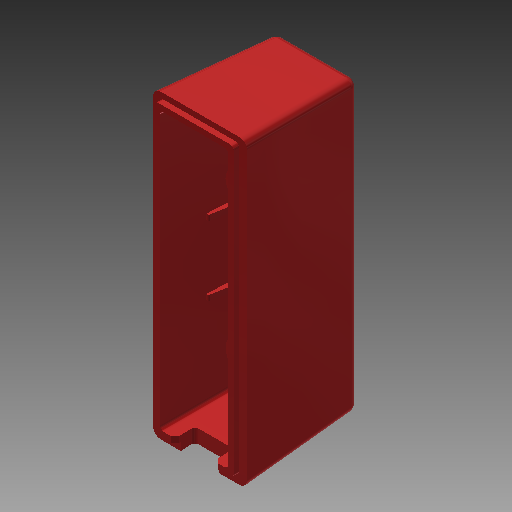
# Autodesk Inventor part: 276-2154
Saved by Autodesk Inventor 2019.4 (Build 234330000, 330)
## iProperties
Category: Sensors
Company: Autodesk Inc.
Created: 2012-03-29
Part Number: 276-2154
Document SubType Name: Modeling
Designer: Autodesk Inc.
Density: 1.06 g/cm^3
Material: ABS Plastic
Catalog Web Link: http://www.vexrobotics.com/276-2154.html
Vendor: VEX
Mass: 3.18655 g
Surface Area: 37.1794 cm^2
Volume: 3.00618 cm^3
Appearance: 浅红色
Author: Autodesk Inc.
Autodesk Inventor part; units mm, degrees
ref_plane "YZ Plane" through (0, 0, 0) normal (1, 0, 0) x (0, 1, 0)
ref_plane "XY Plane" through (0, 0, 0) normal (0, 0, 1) x (1, 0, 0)
sketch "Sketch1" plane through (0, 0, 0) normal (0, 0, 1) x (1, 0, 0)
  line L0 (-1.6366, -1.7521) -> (10.53, -1.7521)
  line L1 (6.89, -1.7521) -> (10.53, -1.7521)
  line L2 (10.53, 37.2479) -> (10.53, -1.7521)
  line L3 (10.53, 37.2479) -> (-1.6366, 37.2479)
  line L4 (-1.6366, 37.2479) -> (-1.6366, -1.7521)
  point P0 (4.4467, 17.7479)
  point P1 (4.4467, 37.2479)
  dimension "d19" = 12.1666
  constraints: 10 end point, 2 horizontal, 1 midpoint, 1 vertical, 1 vertical alignment
  measures "d19" distance between parallel lines of L2 L4
extrude "Extrusion1" add sketch "Sketch1" against normal blind 15.1892 draft -3
fillet "Fillet1" radius 0.9906 8 edges at (-1.2386, 36.8499, -7.5946) (4.4467, -0.956, -15.1892) (-0.8406, 17.7479, -15.1892) (4.4467, 36.4519, -15.1892) (10.132, 36.8499, -7.5946) (9.734, 17.7479, -15.1892) (10.132, -1.354, -7.5946) (-1.2386, -1.354, -7.5946)
sketch "Sketch2" plane through (0, 0, 0) normal (0, 0, 1) x (1, 0, 0)
  line L0 (-0.7514, -1.7426) -> (1.89, -1.7426)
  line L1 (-0.734, -0.7266) -> (-0.734, 36.5367)
  line L2 (-0.734, 36.5367) -> (9.514, 36.5367)
  line L3 (9.514, 36.5367) -> (9.514, -0.7266)
  line L4 (9.514, -0.7266) -> (-0.734, -0.7266)
  line L5 (6.89, -1.7426) -> (9.5314, -1.7426)
  ellipse E0 centre (9.5286, -0.7413) end of major axis (8.8196, -0.0322) minor radius 1 (9.5314, -1.7426) -> (10.53, -0.744) ccw
  line L6 (10.53, 36.2587) -> (10.53, -0.744)
  ellipse E1 centre (9.5286, 36.256) end of major axis (10.2377, 36.965) minor radius 1 (10.53, 36.2587) -> (9.5314, 37.2574) ccw
  line L7 (9.5314, 37.2574) -> (-0.7514, 37.2574)
  ellipse E2 centre (-0.7486, 36.256) end of major axis (-1.4577, 36.965) minor radius 1 (-0.7514, 37.2574) -> (-1.75, 36.2587) ccw
  line L8 (-1.75, 36.2587) -> (-1.75, -0.744)
  ellipse E3 centre (-0.7486, -0.7413) end of major axis (-0.0396, -0.0322) minor radius 1 (-1.75, -0.744) -> (-0.7514, -1.7426) ccw
  ellipse E4 centre (9.538, -0.7601) end of major axis (10.2404, -1.4625) minor radius 0.9906 (9.5408, -1.7521) -> (10.53, -0.7628) ccw projected
  line L9 (10.53, -0.7628) -> (10.53, 36.2587) projected
  ellipse E5 centre (9.538, 36.256) end of major axis (10.2404, 36.9584) minor radius 0.9906 (10.53, 36.2587) -> (9.5408, 37.2479) ccw projected
  line L10 (9.5408, 37.2479) -> (-0.6474, 37.2479) projected
  ellipse E6 centre (-0.6446, 36.256) end of major axis (-1.347, 36.9584) minor radius 0.9906 (-0.6474, 37.2479) -> (-1.6366, 36.2587) ccw projected
  line L11 (-1.6366, 36.2587) -> (-1.6366, -0.7628) projected
  ellipse E7 centre (-0.6446, -0.7601) end of major axis (-1.347, -1.4625) minor radius 0.9906 (-1.6366, -0.7628) -> (-0.6474, -1.7521) ccw projected
  line L12 (-0.6474, -1.7521) -> (9.5408, -1.7521) projected
  line L13 (8.8028, 35.8255) -> (-0.0228, 35.8255)
  line L14 (-0.0228, 35.8255) -> (-0.0228, -0.0154)
  line L15 (-0.0228, -0.0154) -> (8.8028, -0.0154)
  line L16 (8.8028, -0.0154) -> (8.8028, 35.8255)
  point P0 (4.3806, 17.7574)
  dimension "d3" = 0.7112
  dimension "d6" = 1.016
  dimension "d7" = 1.016
  dimension "d8" = 1.016
  dimension "d9" = 0.7112
  constraints: 26 end point, 1 collinear, 23 other
  measures "d3" distance between parallel lines of L2 L13
  measures "d6" distance between parallel lines of L6 L3
  measures "d7" distance between parallel lines of L8 L1
  measures "d8" distance between parallel lines of L5 L4
  measures "d9" distance between parallel lines of L10 L2
extrude "Extrusion3" add sketch "Sketch2" along normal blind 0.7112 contours L1 L2 L3 L4 | L16 L15 L14 L13
sketch "Sketch3" plane through (0, 0, 0.7112) normal (0, 0, 1) x (1, 0, 0)
  line L0 (8.8028, 35.8255) -> (-0.0228, 35.8255) projected
  line L1 (-0.0228, 35.8255) -> (-0.0228, -0.0154) projected
  line L2 (8.8028, -0.0154) -> (8.8028, 35.8255) projected
  line L3 (-0.0228, -0.0154) -> (8.8028, -0.0154) projected
  point P0 (0, 0)
extrude "Extrusion4" cut sketch "Sketch3" against normal blind 13.6906 draft -3
fillet "Fillet4" radius 1.4986 2 edges at (4.39, 35.108, -12.9794) (4.39, 0.702, -12.9794)
fillet "Fillet6" radius 0.508 4 edges at (9.514, -0.7266, 0.3556) (-0.734, -0.7266, 0.3556) (9.514, 36.5367, 0.3556) (-0.734, 36.5367, 0.3556)
ref_plane "Work Plane1" through (0, 0, -5.2832) normal (0, 0, 1) x (1, 0, 0)
sketch "Sketch4" plane through (0, 0, -5.2832) normal (0, 0, 1) x (1, 0, 0)
  circle A0 centre (4.4422, 26.4337) radius 1.5321 projected
  circle A1 centre (4.4422, 7.4345) radius 1.5321 projected
  circle A2 centre (4.4422, 26.4337) radius 1.9939
  circle A3 centre (4.4422, 7.4345) radius 1.9939
  point P0 (0, 0)
  dimension "d21" = 3.9878
  constraints: 2 centre point, 2 coincident, 1 equal radius
  measures "d21" diameter of A2
extrude "Extrusion5" add sketch "Sketch4" against normal up to next contours A0 | A1 | A2 | A3
sketch "Sketch5" plane through (4.4422, 7.4345, -5.2832) normal (0, 0, 1) x (1, 0, 0)
  circle A0 centre (0, 0) radius 1.9939 projected
  circle A1 centre (0, 18.9992) radius 1.9939 projected
  point P0 (-4.4422, -7.4345)
hole "Hole1" at (4.4422, 7.4345, -5.2832) at (4.4422, 26.4337, -5.2832) direction (0, 0, -1) diameter 1.7018 depth 8.2042
ref_plane "Work Plane2" through (0, 0, -7.9756) normal (0, 0, 1) x (1, 0, 0)
sketch "Sketch7" plane through (0, 0, -7.9756) normal (0, 0, 1) x (1, 0, 0)
  circle A0 centre (4.4422, 26.4337) radius 0.8509 projected
  line L0 (-0.0228, -0.0154) -> (-0.0228, 35.8255) projected
  line L1 (8.8028, 35.8255) -> (8.8028, -0.0154) projected
  circle A1 centre (4.4422, 26.4337) radius 1.9939 projected
  line L2 (3.709, 24.5795) -> (-0.0228, 24.5795)
  line L3 (-0.0228, 23.7413) -> (8.8028, 23.7413)
  line L4 (5.1754, 24.5795) -> (8.8028, 24.5795)
  ellipse E0 centre (8.1638, 2.1242) end of major axis (8.1638, 0.6256) minor radius 0.0785 (8.0853, 2.1242) -> (8.1597, 0.6276) ccw projected
  line L5 (8.8028, -0.0154) -> (8.1597, 0.6276) projected
  line L6 (8.8028, 35.8255) -> (8.1597, 35.1825) projected
  ellipse E1 centre (8.1638, 33.6859) end of major axis (8.1638, 32.1873) minor radius 0.0785 (8.1597, 35.1825) -> (8.0853, 33.6859) ccw projected
  line L7 (8.0853, 2.1242) -> (8.0853, 33.6859) projected
  ellipse E2 centre (0.6162, 2.1242) end of major axis (0.6162, 3.6228) minor radius 0.0785 (0.6203, 0.6276) -> (0.6947, 2.1242) ccw projected
  line L8 (0.6947, 33.6859) -> (0.6947, 2.1242) projected
  ellipse E3 centre (0.6162, 33.6859) end of major axis (0.6162, 35.1845) minor radius 0.0785 (0.6947, 33.6859) -> (0.6203, 35.1825) ccw projected
  line L9 (-0.0228, 35.8255) -> (0.6203, 35.1825) projected
  line L10 (-0.0228, -0.0154) -> (0.6203, 0.6276) projected
  point P0 (0, 0)
  dimension "d32" = 1.8542
  dimension "d33" = 0.8382
  constraints: 6 end point, 4 point on line, 2 parallel, 2 point on circle, 1 collinear, 4 other
  measures "d32" distance from line of L2 A0.centre
  measures "d33" distance between parallel lines of L3 L2
extrude "Extrusion6" add sketch "Sketch7" against normal up to next draft 1 contours A0 | L0 L2 L8 L3 | L8 L2 A1 L4 L7 L3 | L7 L4 L1 L3 | A1
ref_plane "Work Plane4" through (4.4422, 16.9341, -5.2832) normal (0, 1, 0) x (0, 0, -1)
ref_plane "Work Plane3" through (4.4422, 7.4345, -5.2832) normal (0, 1, 0) x (0, 0, -1)
mirror "Mirror1" about plane through (4.4422, 16.9341, -5.2832) normal (0, 1, 0) of "Extrusion6"
fillet "Fillet7" radius 0.508 12 edges at (0.6731, 1.0926, -12.5678) (0.6947, 5.6628, -12.9794) (0.2987, 0.3061, -5.424) (0.6947, 29.1764, -12.9794) (0.6731, 34.7175, -12.5678) (0.2987, 35.504, -5.424) (8.0853, 29.1764, -12.9794) (8.1069, 34.7175, -12.5678) (8.4813, 35.504, -5.424) (8.0853, 5.6628, -12.9794) (8.1069, 1.0926, -12.5678) (8.4813, 0.3061, -5.424)
sketch "Sketch10" plane through (0, 0, -12.9794) normal (0, 0, 1) x (1, 0, 0)
  line L0 (0.6947, 23.654) -> (0.6947, 10.2142) projected
  line L1 (1.088, 10.2142) -> (7.692, 10.2142)
  line L2 (7.692, 10.2142) -> (7.692, 23.654)
  line L3 (7.692, 23.654) -> (1.088, 23.654)
  line L4 (1.088, 23.654) -> (1.088, 10.2142)
  line L5 (0.4325, 10.1269) -> (8.3475, 10.1269) projected
  point P0 (0, 0)
  point P1 (1.088, 16.9341)
  point P2 (0.6947, 16.9341)
  point P3 (4.39, 10.2142)
  point P4 (4.39, 10.1269)
  dimension "d47" = 6.604
  constraints: 8 end point, 4 midpoint, 3 parallel, 1 horizontal, 1 horizontal alignment, 1 perpendicular, 1 vertical alignment
  measures "d47" distance between parallel lines of L4 L2
sketch "Sketch11" plane through (0, 0, -15.1892) normal (0, 0, -1) x (-1, 0, 0)
  line L0 (-0.6947, 10.2142) -> (-8.0853, 10.2142) projected
  line L1 (-8.0853, 10.2142) -> (-8.0853, 23.654) projected
  line L2 (-8.0853, 23.654) -> (-0.6947, 23.654) projected
  line L3 (-0.6947, 23.654) -> (-0.6947, 10.2142) projected
  line L4 (-1.088, 10.2285) -> (-7.692, 10.2285)
  line L5 (-7.692, 10.2285) -> (-7.692, 23.6397)
  line L6 (-7.692, 23.6397) -> (-1.088, 23.6397)
  line L7 (-1.088, 23.6397) -> (-1.088, 10.2285)
  point P0 (0, 0)
  point P1 (-4.39, 10.2285)
  point P2 (-4.39, 10.2142)
  point P3 (-7.692, 16.9341)
  point P4 (-8.0853, 16.9341)
  dimension "d44" = 6.604
  dimension "d45" = 13.4112
  constraints: 8 end point, 4 midpoint, 2 parallel, 1 horizontal, 1 horizontal alignment, 1 perpendicular, 1 vertical alignment
  measures "d44" distance of L5.end L6.end
  measures "d45" distance of L4.end L5.end
loft "Loft1" cut profiles "Sketch10", "Sketch11" contours all / L4 L5 L6 L7
ref_plane "Work Plane6" through (7.692, 11.8398, -12.9794) normal (0, -1, 0) x (1, 0, 0)
ref_plane "Work Plane5" through (7.692, 10.2142, -12.9794) normal (0, -1, 0) x (1, 0, 0)
sketch "Sketch13" plane through (7.692, 11.8398, -12.9794) normal (0, -1, 0) x (1, 0, 0)
  line L0 (0.3933, 0) -> (0.6555, 5.0038) projected
  line L1 (0, 0) -> (0.3933, 0) projected
  line L2 (0, 0) -> (0, -2.2098) projected
  line L3 (0, 0) -> (0, 8.0264)
  line L4 (1.1108, 13.6906) -> (0.4677, 1.4202) projected
  line L5 (0, 8.0264) -> (0.814, 8.0264)
  point P0 (-7.692, 12.9794)
  dimension "d64" = 8.0264
  dimension "d71" = 0.3933
  constraints: 4 end point, 1 perpendicular, 1 point on line, 1 vertical
  measures "d64" distance of L1.start L3.end
  measures "d71" distance of L1.start L0.start
extrude "Extrusion9" add sketch "Sketch13" against normal blind 0.7112
sketch "Sketch14" plane through (7.692, 12.551, -12.9794) normal (0, 1, 0) x (1, 0, 0)
  line L0 (0, -8.0264) -> (0, 0) projected
  line L1 (0.814, -8.0264) -> (0, -8.0264) projected
  line L2 (0, -5.1816) -> (0.508, -8.0264)
  point P0 (-7.692, -12.9794)
  dimension "d67" = 0.508
  dimension "d68" = 2.8448
  constraints: 2 end point, 2 point on line
  measures "d67" distance of L2.end L0.start
  measures "d68" vertical distance of L2.start L2.end
extrude "Extrusion10" cut sketch "Sketch14" against normal up to next
fillet "Fillet9" radius 0.254 1 edges at (8.2, 12.1954, -4.953)
pattern_linear "Rectangular Pattern1" count 2 spacing 8.9916 along (0, 1, 0) of "Extrusion9", "Extrusion10", "Fillet9"
ref_plane "Work Plane7" through (4.39, -0.0154, 0.7112) normal (-1, 0, 0) x (0, -1, 0)
mirror "Mirror2" about plane through (4.39, -0.0154, 0.7112) normal (-1, 0, 0) of "Extrusion9", "Extrusion10", "Fillet9", "Rectangular Pattern1"
ref_plane "Work Plane8" through (10.53, 37.2479, 0) normal (0, 1, 0) x (-1, 0, 0)
ref_plane "Work Plane9" through (-1.6366, -1.7521, 0) normal (0, 1, 0) x (1, 0, 0)
sketch "Sketch16" plane through (-1.6366, -1.7521, 0) normal (0, 1, 0) x (1, 0, 0)
  line L0 (10.6426, -0.7112) -> (1.4106, -0.7112) projected
  line L1 (8.5852, -0.7112) -> (8.5852, 1.3034)
  line L2 (8.0852, 1.8034) -> (4.0814, 1.8034)
  line L3 (3.5814, 1.3034) -> (3.5814, -0.7112)
  arc A0 (8.5852, 1.3034) -> (8.0852, 1.8034) centre (8.0852, 1.3034) ccw
  arc A1 (4.0814, 1.8034) -> (3.5814, 1.3034) centre (4.0814, 1.3034) ccw
  line L4 (11.1774, 0) -> (10.4305, 14.2504) projected
  line L5 (0.9892, 0) -> (11.1774, 0) projected
  line L6 (1.7361, 14.2504) -> (0.9892, 0) projected
  line L7 (10.4305, 14.2504) -> (1.7361, 14.2504) projected
  point P0 (1.6366, 0)
  point P1 (6.0833, 1.8034)
  point P2 (6.0266, -0.7112)
  point P3 (6.0833, 0)
  dimension "d89" = 0.5
  dimension "d90" = 5.0038
  dimension "d91" = 2.5146
  constraints: 6 end point, 4 point on circle, 4 tangent, 3 midpoint, 2 centre point, 2 perpendicular, 2 point on line, 1 equal radius, 1 parallel, 1 vertical alignment
  measures "d89" radius of A0
  measures "d90" distance between parallel lines of L3 L1
  measures "d91" distance between parallel lines of L2 L0
extrude "Extrusion12" cut sketch "Sketch16" along normal up to next contours L0 L3 L5 L1 | L5 L3 A1 L2 A0 L1
chamfer "Chamfer3" distance 0.508 angle 45 2 edges at (6.9486, -0.371, 0.7112) (1.9448, -0.371, 0.7112)
thread "Thread1" size "M2x0.4" class "6H" standard "ANSI Metric M Profile" full length
thread "Thread2" size "1-64 UNC" class "2B" standard "ANSI Unified Screw Threads" full length
equation "\"d7\" = d6"
equation "\"d8\" = d6"
equation "\"d9\" = d3"
body "Solid1"
